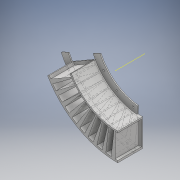
# Autodesk Inventor part: stator-sextant-v2
Saved by Autodesk Inventor 2018 (Build 220112000, 112)
## iProperties
Created: 2025-03-12
Part Number: stator-sextant-v2
Material: Generic
Document SubType Name: Modeling
Designer: neo
Density: 1 g/cm^3
Appearance: Default
Author: neo
Autodesk Inventor part; units mm, degrees
ref_plane "YZ Plane" through (0, 0, 0) normal (1, 0, 0) x (0, 1, 0)
ref_plane "XZ Plane" through (0, 0, 0) normal (0, 1, 0) x (-1, 0, 0)
ref_plane "XY Plane" through (0, 0, 0) normal (0, 0, 1) x (1, 0, 0)
sketch "Sketch4" plane through (0, 0, 0) normal (0, 1, 0) x (-1, 0, 0)
  circle A0 centre (0, 0) radius 104
  circle A1 centre (0, 0) radius 157.5
  line L0 (0, 0) -> (0, -372.6327)
  line L1 (5.25, -107) -> (-5.25, -107)
  line L2 (-5.25, -107) -> (-5.25, -153.5)
  line L3 (-5.25, -153.5) -> (5.25, -153.5)
  line L4 (5.25, -153.5) -> (5.25, -107)
  line L5 (0, -104) -> (55.222, -104) construction
  line L6 (0, -157.5) -> (46.4746, -157.5) construction
  dimension "d16" = 208
  dimension "d12" = 46.5
  dimension "d13" = 3
  dimension "d14" = 10.5
  dimension "d15" = 4
  constraints: 14 end point, 3 horizontal, 2 coincident, 2 parallel, 2 perpendicular, 2 point on line, 2 vertical alignment, 1 vertical, 5 other
  measures "d12" distance of L3.end L1.start
  measures "d13" distance between parallel lines of L5 L1
  measures "d14" distance between parallel lines of L2 L4
  measures "d15" distance between parallel lines of L3 L6
extrude "Extrusion3" add sketch "Sketch4" along normal blind 46.5 contours A1 | L1 L4 L3 L0 | L0 L3 L2 L1
extrude "Extrusion4" cut sketch "Sketch4" along normal through all contours L1 L4 L3 L0 | L0 L3 L2 L1
pattern_circular "Circular Pattern1" count 54 over 360 about axis through (0, 0, 0) along (0, 1, 0) of "Extrusion4"
sketch "Sketch5" plane through (0, 46.5, 0) normal (0, 1, 0) x (1, 0, 0)
  line L0 (0, 0) -> (0, 197.0363)
  line L1 (0, 0) -> (-170.6385, 98.5182)
  arc A0 (-170.6385, 98.5182) -> (0, 197.0363) centre (0, 0) ccw
  dimension "d24" = 60
  constraints: 4 end point, 2 point on circle, 1 centre point, 1 coincident, 1 vertical
  measures "d24" angle of L0 L1
extrude "Extrusion5" cut sketch "Sketch5" against normal through all
sketch "Sketch6" plane through (0, 46.5, 0) normal (0, 1, 0) x (1, 0, 0)
  line L0 (-92.6647, 53.5) -> (-90.0666, 52) construction
  arc A0 (0, 104) -> (-90.0666, 52) centre (0, 0) ccw construction
  line L1 (0, 104) -> (0, 107) construction
  line L2 (0, 107) -> (-5.25, 107) construction
  line L3 (-5.25, 107) -> (-5.25, 153.5) construction
  line L4 (-5.25, 153.5) -> (0, 153.5) construction
  line L5 (0, 153.5) -> (0, 157.5) construction
  arc A1 (0, 157.5) -> (-136.399, 78.75) centre (0, 0) ccw construction
  line L6 (-136.399, 78.75) -> (-132.9349, 76.75) construction
  line L7 (-132.9349, 76.75) -> (-130.3099, 81.2966) construction
  line L8 (-130.3099, 81.2966) -> (-90.0397, 58.0466) construction
  line L9 (-90.0397, 58.0466) -> (-92.6647, 53.5) construction
  line L10 (-12.6058, 153.0716) -> (-7.2074, 106.886) construction
  line L11 (-7.2074, 106.886) -> (-17.6364, 105.667) construction
  line L12 (-17.6364, 105.667) -> (-23.0348, 151.8526) construction
  line L13 (-23.0348, 151.8526) -> (-12.6058, 153.0716) construction
  line L14 (-30.2911, 150.5731) -> (-19.5674, 105.3265) construction
  line L15 (-19.5674, 105.3265) -> (-29.7844, 102.9051) construction
  line L16 (-29.7844, 102.9051) -> (-40.508, 148.1517) construction
  line L17 (-40.508, 148.1517) -> (-30.2911, 150.5731) construction
  line L18 (-47.5667, 146.0384) -> (-31.6628, 102.3427) construction
  line L19 (-31.6628, 102.3427) -> (-41.5295, 98.7515) construction
  line L20 (-41.5295, 98.7515) -> (-57.4335, 142.4472) construction
  line L21 (-57.4335, 142.4472) -> (-47.5667, 146.0384) construction
  line L22 (-64.1991, 139.5288) -> (-43.3299, 97.9749) construction
  line L23 (-43.3299, 97.9749) -> (-52.7131, 93.2625) construction
  line L24 (-52.7131, 93.2625) -> (-73.5822, 134.8164) construction
  line L25 (-73.5822, 134.8164) -> (-64.1991, 139.5288) construction
  line L26 (-79.9633, 131.1323) -> (-54.4111, 92.2821) construction
  line L27 (-54.4111, 92.2821) -> (-63.1838, 86.5123) construction
  line L28 (-63.1838, 86.5123) -> (-88.7359, 125.3625) construction
  line L29 (-88.7359, 125.3625) -> (-79.9633, 131.1323) construction
  line L30 (-94.6462, 120.9625) -> (-64.7565, 85.3414) construction
  line L31 (-64.7565, 85.3414) -> (-72.8, 78.5921) construction
  line L32 (-72.8, 78.5921) -> (-102.6896, 114.2132) construction
  line L33 (-102.6896, 114.2132) -> (-94.6462, 120.9625) construction
  line L34 (-108.0491, 109.1568) -> (-74.2262, 77.2466) construction
  line L35 (-74.2262, 77.2466) -> (-81.4317, 69.6091) construction
  line L36 (-81.4317, 69.6091) -> (-115.2546, 101.5194) construction
  line L37 (-115.2546, 101.5194) -> (-108.0491, 109.1568) construction
  line L38 (-119.9908, 95.875) -> (-82.6921, 68.1071) construction
  line L39 (-82.6921, 68.1071) -> (-88.9623, 59.6848) construction
  line L40 (-88.9623, 59.6848) -> (-126.261, 87.4527) construction
  line L41 (-126.261, 87.4527) -> (-119.9908, 95.875) construction
  arc A2 (0, 172.5) -> (-149.3894, 86.25) centre (0, 0) ccw
  line L42 (0, 104) -> (0, 172.5)
  line L43 (0, 0) -> (-90.0666, 52) construction
  arc A3 (0, 89) -> (-77.0763, 44.5) centre (0, 0) ccw
  line L44 (0, 89) -> (0, 172.5)
  line L45 (-77.0763, 44.5) -> (-149.3894, 86.25)
  arc A4 (0, 104) -> (-90.0666, 52) centre (0, 0) ccw projected
  arc A5 (0, 157.5) -> (-136.399, 78.75) centre (0, 0) ccw projected
  line L46 (0, 0) -> (-41.5132, 235.433) construction
  arc A6 (0, 96.5) -> (-89.9528, 34.9391) centre (0, 0) ccw construction
  arc A7 (6.0545, 164.8889) -> (-149.3539, 70.1315) centre (0, 0) ccw construction
  circle A8 centre (-16.757, 95.0339) radius 1.75
  circle A9 centre (-28.6519, 162.4933) radius 1.75
  circle A10 centre (-48.25, 83.5715) radius 1.75
  circle A11 centre (-82.5, 142.8942) radius 1.75
  circle A12 centre (-73.9233, 62.029) radius 1.75
  circle A13 centre (-126.3973, 106.06) radius 1.75
  dimension "d27" = 15
  dimension "d29" = 15
  dimension "d31" = 60
  dimension "d32" = 15
  dimension "d33" = 10
  dimension "d34" = 7.5
  dimension "d35" = 7.5
  dimension "d36" = 3.5
  dimension "d37" = 3.5
  dimension "d40" = 40
  constraints: 10 centre point, 10 end point, 10 point on circle, 4 point on line, 3 coincident, 2 vertical, 1 collinear, 9 other
  measures "d27" radial gap between concentric circles of A1 A2
  measures "d29" radial gap between concentric circles of A0 A3
  measures "d31" angle of L44 L43
  measures "d32" distance of L42.end L5.end
  measures "d33" angle of L42 L46
  measures "d34" radial gap between concentric circles of A7 A2
  measures "d35" radial gap between concentric circles of A3 A6
  measures "d36" diameter of A8
  measures "d37" diameter of A9
extrude "Extrusion6" add sketch "Sketch6" along normal blind 2
sketch "Sketch7" plane through (0, 0, -153.5) normal (1, 0, 0) x (0, 0, -1)
  line L0 (-49.5, 0) -> (-49.5, 46.5) projected
  line L1 (-46.5, 0) -> (-49.5, 0) projected
  line L2 (-46.5, 46.5) -> (-46.5, 0) projected
  line L3 (-46.5, 46.5) -> (0, 46.5) projected
  line L4 (0, 0) -> (0, 46.5) projected
  line L5 (4, 0) -> (0, 0) projected
  line L6 (4, 46.5) -> (4, 0) projected
  line L7 (4, 46.5) -> (19, 46.5) projected
  line L8 (19, 46.5) -> (19, 48.5) projected
  line L9 (-64.5, 48.5) -> (19, 48.5) projected
  line L10 (-64.5, 46.5) -> (-64.5, 48.5) projected
  line L11 (-64.5, 46.5) -> (-49.5, 46.5) projected
  line L12 (19, 48.5) -> (-67.25, 48.5) projected
  line L13 (4, 46.5) -> (19, 46.5) projected
  line L14 (19, 48.5) -> (4, 48.5)
  line L15 (4, 48.5) -> (4, 46.5)
  line L16 (4, 46.5) -> (19, 46.5)
  line L17 (19, 46.5) -> (19, 48.5)
  line L18 (-101.5, 46.5) -> (-49.5, 46.5) projected
  line L19 (-109, 48.5) -> (-64.5, 48.5) projected
  line L20 (-49.5, 46.5) -> (-64.5, 46.5)
  line L21 (-64.5, 46.5) -> (-64.5, 48.5)
  line L22 (-64.5, 48.5) -> (-49.5, 48.5)
  line L23 (-49.5, 48.5) -> (-49.5, 46.5)
  line L24 (-153.5, -9.7) -> (-153.5, 58.2) projected
  point P0 (-153.5, 0)
  constraints: 16 end point, 4 parallel, 2 horizontal, 2 perpendicular
revolve "cut 5 deg" cut sketch "Sketch7" angle 5 about axis through (0, 0, 0) along (0, 1, 0) contours L11 L10 L9 L23 | L9 L8 L7 L15
sketch "Sketch8" plane through (-92.6647, 0, -53.5) normal (-0.5, 0, 0.8660254) x (0.8660254, 0, 0.5)
  line L0 (0, 0) -> (0, 46.5) projected
  line L1 (3, 0) -> (0, 0) projected
  line L2 (3, 46.5) -> (3, 0) projected
  line L3 (3, 46.5) -> (18, 46.5) projected
  line L4 (18, 46.5) -> (18, 48.5) projected
  line L5 (-65.5, 48.5) -> (18, 48.5) projected
  line L6 (-65.5, 46.5) -> (-65.5, 48.5) projected
  line L7 (-65.5, 46.5) -> (-50.5, 46.5) projected
  line L8 (-50.5, 0) -> (-50.5, 46.5) projected
  line L9 (-46.5, 0) -> (-50.5, 0) projected
  line L10 (-46.5, 46.5) -> (-46.5, 0) projected
  line L11 (-46.5, 46.5) -> (0, 46.5) projected
  line L12 (-65.5, 48.5) -> (18, 48.5) projected
  line L13 (18, 46.5) -> (3, 46.5)
  line L14 (3, 46.5) -> (3, 48.5)
  line L15 (3, 48.5) -> (18, 48.5)
  line L16 (18, 48.5) -> (18, 46.5)
  line L17 (-65.5, 46.5) -> (-50.5, 46.5) projected
  line L18 (8.0581, 48.5) -> (-65.5, 48.5) projected
  line L19 (-50.5, 46.5) -> (-65.5, 46.5)
  line L20 (-65.5, 46.5) -> (-65.5, 48.5)
  line L21 (-65.5, 48.5) -> (-50.5, 48.5)
  line L22 (-50.5, 48.5) -> (-50.5, 46.5)
  line L23 (107, -9.7) -> (107, 58.2) projected
  point P0 (107, 0)
  constraints: 16 end point, 4 parallel, 2 horizontal, 2 perpendicular, 1 point on line
revolve "Revolution2" add sketch "Sketch8" angle 5 about axis through (0, 0, 0) along (0, 1, 0) contours L14 L5 L4 L3 | L22 L7 L6 L5
equation "\"platesize\" = 46"
body "Solid2"
